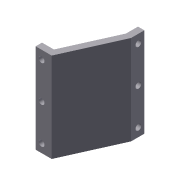
# Autodesk Inventor part: Trunk
Saved by Autodesk Inventor 2011 (Build 150239000, 239)
## iProperties
Created: 2010-11-22
Part Number: Trunk
Document SubType Name: Modeling
Designer: Milton
Density: 2.71 g/cm^3
Mass: 13.1719 g
Surface Area: 38.8137 cm^2
Volume: 4.86049 cm^3
Material: Aluminum-6061
Author: Milton
Autodesk Inventor part; units mm, degrees
ref_plane "YZ Plane" through (0, 0, 0) normal (1, 0, 0) x (0, 1, 0)
ref_plane "XZ Plane" through (0, 0, 0) normal (0, 1, 0) x (-1, 0, 0)
ref_plane "XY Plane" through (0, 0, 0) normal (0, 0, 1) x (1, 0, 0)
sketch "Sketch1" plane through (0, 0, 0) normal (0, 0, 1) x (1, 0, 0)
  line L0 (22.7021, 34.3404) -> (19.7021, 34.3404)
  line L1 (19.7021, 34.3404) -> (19.7021, 28.7404)
  line L2 (19.7021, 28.7404) -> (9.3021, 5.3404)
  line L3 (22.7021, 28.1038) -> (11.2517, 2.3404)
  line L4 (9.3021, 5.3404) -> (3.7021, 5.3404)
  line L5 (3.7021, 5.3404) -> (3.7021, 2.3404)
  line L6 (22.7021, 34.3404) -> (22.7021, 28.1038)
  line L7 (3.7021, 2.3404) -> (11.2517, 2.3404)
  point P0 (0, 0)
  dimension "d0" = 3
  dimension "d1" = 3
  dimension "d2" = 32
  dimension "d3" = 19
  dimension "d4" = 5.6
  dimension "d5" = 5.6
  dimension "d6" = 3
  constraints: 16 end point, 2 vertical, 1 parallel
  measures "d0" distance of L0.start L0.end
  measures "d1" distance of L4.end L5.end
  measures "d2" distance between parallel lines of L7 L0
  measures "d3" distance between parallel lines of L6 L5
  measures "d4" distance of L0.end L1.end
  measures "d5" distance of L2.end L4.end
  measures "d6" distance between parallel lines of L3 L2
extrude "Extrusion1" add sketch "Sketch1" along normal blind 42
sketch "Sketch2" plane through (3.7021, 5.3404, 0) normal (0, 1, 0) x (1, 0, 0)
  line L0 (0, -42) -> (5.6, -42) projected
  circle A0 centre (2.8, -4) radius 1.35
  circle A1 centre (2.8, -21) radius 1.35
  circle A2 centre (2.8, -38) radius 1.35
  point P0 (-3.7021, 0)
  dimension "d9" = 2.7
  dimension "d10" = 2.7
  dimension "d11" = 2.7
  dimension "d12" = 17
  dimension "d13" = 17
  dimension "d14" = 4
  constraints: 3 centre point
  measures "d9" diameter of A0
  measures "d10" diameter of A1
  measures "d11" diameter of A2
  measures "d12" distance of A1.centre A0.centre
  measures "d13" distance of A2.centre A1.centre
  measures "d14" distance from line of L0 A2.centre
extrude "Extrusion2" cut sketch "Sketch2" against normal through all
sketch "Sketch3" plane through (19.7021, 28.7404, 0) normal (-1, 0, 0) x (0, 0, 1)
  line L0 (0, 5.6) -> (42, 5.6) projected
  line L1 (0, 5.6) -> (0, 0) projected
  circle A0 centre (4, 2.8) radius 1.35
  circle A1 centre (21, 2.8) radius 1.35
  circle A2 centre (38, 2.8) radius 1.35
  point P0 (0, -28.7404)
  dimension "d17" = 2.7
  dimension "d18" = 2.7
  dimension "d19" = 2.7
  dimension "d20" = 17
  dimension "d21" = 17
  dimension "d22" = 4
  dimension "d23" = 2.8
  dimension "d24" = 2.8
  dimension "d25" = 2.8
  constraints: 3 centre point
  measures "d17" diameter of A0
  measures "d18" diameter of A1
  measures "d19" diameter of A2
  measures "d20" distance of A1.centre A0.centre
  measures "d21" distance of A2.centre A1.centre
  measures "d22" distance from line of L1 A0.centre
  measures "d23" distance from line of L0 A0.centre
  measures "d24" distance from line of L0 A1.centre
  measures "d25" distance from line of L0 A2.centre
extrude "Extrusion3" cut sketch "Sketch3" against normal through all
body "Solid1"
